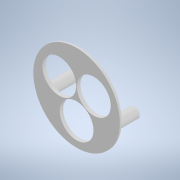
# Autodesk Inventor part: Housing_Front
Saved by Autodesk Inventor 2021 (Build 250183000, 183)
## iProperties
Created: 2026-05-27
Part Number: Housing_Front
Material: Generic
Document SubType Name: Modeling
Designer: Lukas
Density: 1 g/cm^3
Appearance: Default
Author: Lukas
Autodesk Inventor part; units mm, degrees
ref_plane "YZ Plane" through (0, 0, 0) normal (1, 0, 0) x (0, 1, 0)
ref_plane "XZ Plane" through (0, 0, 0) normal (0, 1, 0) x (-1, 0, 0)
ref_plane "XY Plane" through (0, 0, 0) normal (0, 0, 1) x (1, 0, 0)
sketch "Sketch1" plane through (0, 0, 0) normal (0, 0, 1) x (1, 0, 0)
  circle A0 centre (-9.959, 5.75) radius 9.75
  circle A1 centre (0, -11.5) radius 9.75
  circle A2 centre (9.959, 5.75) radius 9.75
  circle A3 centre (0, 0) radius 25
  circle A4 centre (-18, -6) radius 1.4
  circle A5 centre (18, -6) radius 1.4
  circle A6 centre (18, -6) radius 3
  circle A7 centre (-18, -6) radius 3
  circle A8 centre (0, 0) radius 24
  dimension "d0" = 19.918
  dimension "d1" = 5.75
  dimension "d3" = 19.5
  dimension "d4" = 9.959
  dimension "d5" = 17.25
  dimension "d6" = 50
  dimension "d9" = 18
  dimension "d10" = 18
  dimension "d11" = 6
  dimension "d12" = 2.8
  dimension "d13" = 6
  dimension "d20" = 1
  constraints: 9 centre point, 4 coincident, 4 equal radius, 2 horizontal alignment, 1 vertical alignment
  measures "d0" distance of A2.centre A0.centre
  measures "d1" vertical distance of point (0, 0) A0.centre
  measures "d3" diameter of A0
  measures "d4" horizontal distance of point (0, 0) A0.centre
  measures "d5" vertical distance of A0.centre A1.centre
  measures "d6" diameter of A3
  measures "d9" horizontal distance of point (0, 0) A4.centre
  measures "d10" horizontal distance of A5.centre point (0, 0)
  measures "d11" vertical distance of A5.centre point (0, 0)
  measures "d12" diameter of A5
  measures "d13" diameter of A6
  measures "d20" radial gap between concentric circles of A3 A8
extrude "Extrusion1" add sketch "Sketch1" along normal blind 2 contours A3 | A4 | A5 | A6 | A7 | A8
extrude "Extrusion2" add sketch "Sketch1" against normal blind 13.5 contours A6 | A7
chamfer "Chamfer1" distance 1 angle 45 2 edges at (15, -6, 0) (-21, -6, 0)
extrude "Extrusion3" cut sketch "Sketch1" along normal blind 1 contours A3
equation "\"d4\" = 0.5 * d0"
equation "\"d10\" = d9"
body "Solid1"
